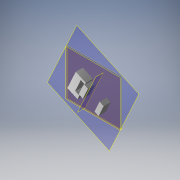
# Autodesk Inventor part: 00_KES_Bluray_Magnet
Saved by Autodesk Inventor 2019 (Build 230136000, 136)
## iProperties
Created: 2019-04-29
Part Number: 00_KES_Bluray_Magnet
Material: Generic
Document SubType Name: Modeling
Designer: diederichbenedict
Density: 1 g/cm^3
Appearance: Chrome - Polished
Author: diederichbenedict
Autodesk Inventor part; units mm, degrees
ref_plane "YZ Plane" through (0, 0, 0) normal (1, 0, 0) x (0, 1, 0)
ref_plane "XZ Plane" through (0, 0, 0) normal (0, 1, 0) x (-1, 0, 0)
ref_plane "XY Plane" through (0, 0, 0) normal (0, 0, 1) x (1, 0, 0)
ref_plane "Work Plane1" through (0, 0, 0) normal (0, 0, 1) x (1, 0, 0)
ref_plane "Work Plane2" through (15.8127, -3.2465, 0) normal (0, 0, -1) x (0.4175, 0.9087, 0)
sketch "Sketch1" plane through (15.8127, -3.2465, 0) normal (0, 0, -1) x (0.4175, 0.9087, 0)
  arc A0 (9.303, -26.8555) -> (8.303, -25.8555) centre (8.303, -26.8555) ccw construction
  line L0 (9.303, -26.8555) -> (9.303, -30) construction
  line L1 (9.303, -30) -> (-16.397, -30) construction
  line L2 (-16.397, -30) -> (-16.397, -20.4723) construction
  arc A1 (-15.397, -19.4723) -> (-16.397, -20.4723) centre (-15.397, -20.4723) ccw construction
  line L3 (-15.397, -19.4723) -> (-13.5347, -19.4723) construction
  arc A2 (-13.5347, -19.4723) -> (-12.5347, -18.4723) centre (-13.5347, -18.4723) ccw construction
  line L4 (-12.5347, -18.4723) -> (-12.5347, 0) construction
  line L5 (-12.5347, 0) -> (-1, 0) construction
  arc A3 (-1, 0) -> (0, 1) centre (-1, 1) ccw construction
  line L6 (0, 1) -> (0, 2) construction
  arc A4 (1, 3) -> (0, 2) centre (1, 2) ccw construction
  line L7 (1, 3) -> (3.5653, 3) construction
  arc A5 (4.5653, 2) -> (3.5653, 3) centre (3.5653, 2) ccw construction
  line L8 (4.5653, 2) -> (4.5653, -24.8555) construction
  arc A6 (4.5653, -24.8555) -> (5.5653, -25.8555) centre (5.5653, -24.8555) ccw construction
  line L9 (5.5653, -25.8555) -> (8.303, -25.8555) construction
  line L10 (2.603, -17.5) -> (2.603, -2) construction
  line L11 (2.603, -2) -> (-10.897, -2) construction
  line L12 (-10.897, -2) -> (-10.897, -17.5) construction
  line L13 (-10.897, -17.5) -> (2.603, -17.5) construction
  circle A7 centre (6.603, -27.5) radius 1 construction
  circle A8 centre (-13.897, -21) radius 1 construction
  circle A9 centre (1.603, 0.5) radius 1 construction
  line L14 (1.603, -19) -> (-7.897, -19)
  line L15 (-7.897, -19) -> (-7.897, -15.5)
  line L16 (-7.897, -15.5) -> (1.603, -15.5)
  line L17 (1.603, -15.5) -> (1.603, -19)
  line L18 (1.603, -2) -> (-7.897, -2)
  line L19 (-7.897, -2) -> (-7.897, -5.5)
  line L20 (-7.897, -5.5) -> (1.603, -5.5)
  line L21 (1.603, -5.5) -> (1.603, -2)
  point P0 (-3.6519, -15.7241)
  dimension "d0" = 9.5
  dimension "d1" = 3.5
  dimension "d2" = 9.5
  dimension "d3" = 3.5
  dimension "d4" = 0
  dimension "d5" = 2.5
  dimension "d6" = 10
  dimension "d7" = 0
  constraints: 16 end point, 4 parallel, 2 horizontal, 2 perpendicular
  measures "d0" distance of L15.end L16.end
  measures "d1" distance of L14.end L15.end
  measures "d2" distance of L20.end L19.end
  measures "d3" distance of L19.end L18.end
  measures "d4" distance from line of A9.centre L21
  measures "d5" distance from line of A9.centre L18
  measures "d6" distance between parallel lines of L20 L16
  measures "d7" distance between parallel lines of L21 L17
extrude "Extrusion1" add sketch "Sketch1" against normal blind 5.5
ref_plane "Work Plane3" through (0, 0, -1) normal (0, 0, -1) x (-1, 0, 0)
sketch "Sketch2" plane through (15.8127, -3.2465, 0) normal (0, 0, -1) x (0.4175, 0.9087, 0)
  line L0 (-11.9051, -26.9073) -> (3.7761, -26.9073)
  line L1 (3.7761, -26.9073) -> (3.7761, -21.7902)
  line L2 (3.7761, -21.7902) -> (-11.9051, -21.7902)
  line L3 (-11.9051, -21.7902) -> (-11.9051, -26.9073)
  line L4 (3.7761, -21.7902) -> (2.1254, -21.7902)
  line L5 (2.1254, -21.7902) -> (2.1254, -18.2413)
  line L6 (2.1254, -18.2413) -> (3.7761, -18.2413)
  line L7 (3.7761, -18.2413) -> (3.7761, -21.7902)
  line L8 (-8.4388, -18.2413) -> (-11.9051, -18.2413)
  line L9 (-11.9051, -18.2413) -> (-11.9051, -21.7902)
  line L10 (-11.9051, -21.7902) -> (-8.4388, -21.7902)
  line L11 (-8.4388, -21.7902) -> (-8.4388, -18.2413)
  point P0 (-3.6519, -15.7241)
  constraints: 24 end point, 6 parallel, 3 horizontal, 3 perpendicular, 1 point on line
extrude "Extrusion2" add sketch "Sketch2" against normal blind 5.5
ref_plane "Arbeitsebene4" through (-2.2914, -8.03, 0) normal (-0.9087, 0.4175, 0) x (0, 0, 1)
body "Solid1"
